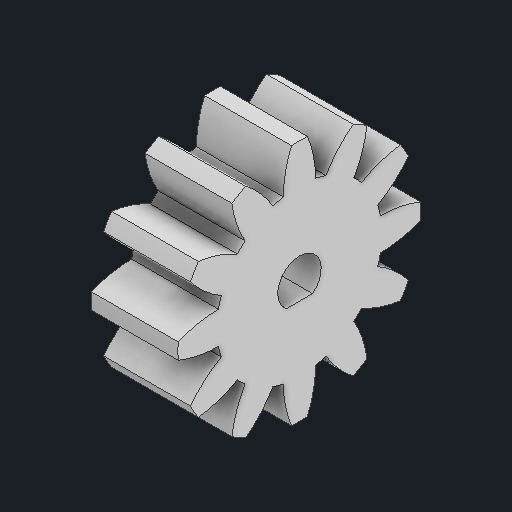
# Autodesk Inventor part: gear1
Saved by Autodesk Inventor 2022 (Build 260153000, 153)
## iProperties
Created: 2022-01-23
Part Number: gear1
Material: Generic
Document SubType Name: Modeling
Designer: gordo
Density: 1 g/cm^3
Appearance: Default
Author: gordo
Autodesk Inventor part; units mm, degrees
ref_plane "YZ Plane" through (0, 0, 0) normal (1, 0, 0) x (0, 1, 0)
ref_plane "XZ Plane" through (0, 0, 0) normal (0, 1, 0) x (-1, 0, 0)
ref_plane "XY Plane" through (0, 0, 0) normal (0, 0, 1) x (1, 0, 0)
sketch "Sketch1" plane through (0, 0, 0) normal (1, 0, 0) x (0, 1, 0)
  circle A0 centre (0, 0) radius 18
  dimension "d0" = 36
  constraints: 1 centre point, 1 coincident
  measures "d0" diameter of A0
extrude "Extrusion1" add sketch "Sketch1" along normal blind 16
sketch "Sketch2" plane through (16, 0, 0) normal (1, 0, 0) x (0, 0, -1)
  circle A0 centre (0, 0) radius 2.5
  line L0 (-1.5, -2) -> (1.5, -2)
  dimension "d3" = 5
  dimension "d7" = 3
  dimension "d8" = 2
  constraints: 2 end point, 1 coincident, 1 horizontal, 3 other
  measures "d7" distance of L0.start L0.end
  measures "d8" distance from line of point (0, 0) L0
extrude "Extrusion2" cut sketch "Sketch2" against normal through all contours A0 L0 picked at (0.6276, -0.7851)
sketch "Sketch3" plane through (16, 0, 0) normal (1, 0, 0) x (0, 0, -1)
  circle A0 centre (0, 0) radius 18
  constraints: 1 centre point, 1 coincident
extrude "Extrusion3" cut sketch "Sketch3" against normal blind 6
sketch "Sketch4" plane through (10, 0, 0) normal (1, 0, 0) x (0, 0, -1)
  circle A0 centre (0, 0) radius 15
  circle A1 centre (0, 0) radius 18
  dimension "d13" = 30
  dimension "d14" = 36
  constraints: 2 centre point, 2 coincident
  measures "d13" diameter of A0
  measures "d14" diameter of A1
extrude "Extrusion4" cut sketch "Sketch4" against normal through all
spur gear teeth "Spur Gear1" teeth 12 pitch diameter 24 tip diameter 27.9657 root diameter 19 face width 10 trims to tip circle yes start plane through (10, 0, 0) normal (1, 0, 0) x (0, 1, 0)
body "Solid1"
